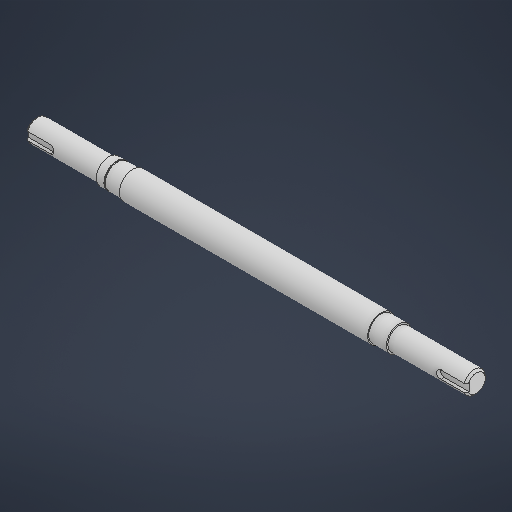
# Autodesk Inventor part: Shaft
Saved by Autodesk Inventor 2026.1 (Build 301233020, 233B)
## iProperties
Created: 2025-10-14
Part Number: Shaft
Material: Generic
Document SubType Name: Modeling
Designer: Alexander
Density: 1 g/cm^3
Appearance: Default
Author: Alexander
Autodesk Inventor part; units mm, degrees
ref_plane "YZ Plane" through (0, 0, 0) normal (1, 0, 0) x (0, 1, 0)
ref_plane "XZ Plane" through (0, 0, 0) normal (0, 1, 0) x (-1, 0, 0)
sketch "Sketch1" plane through (0, 0, 0) normal (0, 0, 1) x (1, 0, 0)
  line L0 (-144.8, -12.5) -> (-137.2, -12.5)
  line L1 (-137.2, -12.5) -> (-137.2, -11.95)
  line L2 (-137.2, -11.95) -> (-136, -11.95)
  line L3 (-136, -11.95) -> (-136, -12.5)
  line L4 (-136, -12.5) -> (-120.8, -12.5)
  line L5 (-120.8, -12.5) -> (-120.8, -13.55)
  line L6 (-120.8, -13.55) -> (127.2, -13.55)
  line L7 (127.2, -13.55) -> (127.2, -12.5)
  line L8 (127.2, -12.5) -> (144.8, -12.5)
  line L9 (144.8, -12.5) -> (144.8, 0)
  line L10 (144.8, 0) -> (-144.8, 0)
  line L11 (-144.8, 0) -> (-144.8, -12.5)
  point P0 (0, 0)
  point P1 (0, 0)
  point P2 (127.2, -13.025)
  dimension "d0" = 12.5
  dimension "d1" = 7.6
  dimension "d2" = 1.2
  dimension "d3" = 0.55
  dimension "d4" = 15.2
  dimension "d5" = 13.55
  dimension "d6" = 11.95
  dimension "d7" = 248
  dimension "d8" = 12.5
  dimension "d9" = 17.6
  constraints: 24 end point, 10 perpendicular, 2 coincident, 2 midpoint, 2 point on line, 1 horizontal
  measures "d0" distance of L10.end L0.start
  measures "d1" distance of L0.start L0.end
  measures "d2" distance of L1.end L2.end
  measures "d3" distance of L0.end L1.end
  measures "d4" distance of L3.end L4.end
  measures "d5" vertical distance of point (0, 0) L5.end
  measures "d6" distance from line of L10 L1.end
  measures "d7" distance of L5.end L6.end
  measures "d8" distance between parallel lines of L10 L8
  measures "d9" distance from line of point (127.2, -13.025) L9
revolve "Revolution1" add sketch "Sketch1" angle 360 about axis through (144.8, 0, 0) along (-1, 0, 0)
sketch "Sketch2" plane through (-144.8, 0, 0) normal (-1, 0, 0) x (0, 0, 1)
  circle A0 centre (0, 0) radius 11
  dimension "d11" = 22
  constraints: 1 centre point, 1 coincident
  measures "d11" diameter of A0
extrude "Extrusion1" add sketch "Sketch2" along normal blind 73
sketch "Sketch3" plane through (144.8, 0, 0) normal (1, 0, 0) x (0, 0, -1)
  point P0 (0, 0)
sketch "Sketch4" plane through (144.8, 0, 0) normal (1, 0, 0) x (0, 0, -1)
  circle A0 centre (0, 0) radius 11
  dimension "d14" = 22
  constraints: 1 centre point, 1 coincident
  measures "d14" diameter of A0
extrude "Extrusion2" add sketch "Sketch4" along normal blind 77.4
ref_plane "Work Plane1" through (-144.8, 0, 11) normal (0, 0, 1) x (1, 0, 0)
sketch "Sketch5" plane through (-144.8, 0, 11) normal (0, 0, 1) x (1, 0, 0)
  line L0 (-73, 11) -> (-73, -11) projected
  line L1 (-73, 4) -> (-48, 4)
  line L2 (-48, 4) -> (-48, -4)
  line L3 (-48, -4) -> (-73, -4)
  line L4 (-73, -4) -> (-73, 4)
  circle A0 centre (-48, 0) radius 4
  line L5 (367, -11) -> (367, 11) projected
  line L6 (367, 4) -> (342, 4)
  line L7 (342, 4) -> (342, -4)
  line L8 (342, -4) -> (367, -4)
  line L9 (367, -4) -> (367, 4)
  circle A1 centre (342, 0) radius 4
  point P0 (144.8, 0)
  point P1 (-73, 0)
  point P2 (367, 0)
  point P3 (367, 0)
  dimension "d17" = 8
  dimension "d18" = 25
  dimension "d19" = 8
  dimension "d20" = 25
  constraints: 16 end point, 5 midpoint, 4 parallel, 2 coincident, 2 horizontal, 2 perpendicular, 2 point on line, 1 horizontal alignment, 6 other
  measures "d17" distance of L1.end L2.end
  measures "d18" distance between parallel lines of L0 L2
  measures "d19" distance of L6.end L7.end
  measures "d20" distance of L6.start L6.end
extrude "Extrusion3" cut sketch "Sketch5" against normal blind 4
chamfer "Chamfer1" distance 2 angle 45 3 edges at (-217.8, 0, -11) (222.2, -10.8101, -2.0351) (222.2, 10.8101, -2.0351)
body "Solid1"
